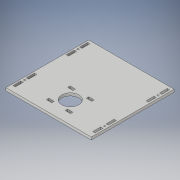
# Autodesk Inventor part: top
Saved by Autodesk Inventor 2018 (Build 220112000, 112)
## iProperties
Created: 2018-04-09
Part Number: top
Material: Generic
Document SubType Name: Modeling
Designer: guita
Density: 1 g/cm^3
Appearance: Default
Author: guita
Autodesk Inventor part; units mm, degrees
ref_plane "YZ Plane" through (0, 0, 0) normal (1, 0, 0) x (0, 1, 0)
ref_plane "XZ Plane" through (0, 0, 0) normal (0, 1, 0) x (-1, 0, 0)
ref_plane "XY Plane" through (0, 0, 0) normal (0, 0, 1) x (1, 0, 0)
sketch "Sketch1" plane through (0, 0, 0) normal (0, 1, 0) x (-1, 0, 0)
  line L0 (0, 0) -> (203.2, 0)
  line L1 (203.2, 0) -> (203.2, -196.85)
  line L2 (203.2, -196.85) -> (0, -196.85)
  line L3 (0, -196.85) -> (0, 0)
  line L4 (0, -196.85) -> (0, -190.5)
  line L5 (3.9624, -190.5) -> (9.525, -190.5)
  line L6 (9.525, -190.5) -> (9.525, -171.45)
  line L7 (9.525, -171.45) -> (3.9624, -171.45)
  circle A0 centre (6.35, -165.1) radius 1.9812
  line L8 (3.9624, -158.75) -> (9.525, -158.75)
  line L9 (9.525, -158.75) -> (9.525, -139.7)
  line L10 (9.525, -139.7) -> (3.9624, -139.7)
  line L11 (3.9624, -12.7) -> (9.525, -12.7)
  line L12 (9.525, -12.7) -> (9.525, -31.75)
  line L13 (9.525, -31.75) -> (3.9624, -31.75)
  circle A1 centre (6.35, -38.1) radius 1.9812
  line L14 (3.9624, -44.45) -> (9.525, -44.45)
  line L15 (9.525, -44.45) -> (9.525, -63.5)
  line L16 (9.525, -63.5) -> (3.9624, -63.5)
  line L17 (199.2376, -190.5) -> (193.675, -190.5)
  line L18 (193.675, -190.5) -> (193.675, -171.45)
  line L19 (193.675, -171.45) -> (199.2376, -171.45)
  circle A2 centre (196.85, -165.1) radius 1.9812
  line L20 (199.2376, -158.75) -> (193.675, -158.75)
  line L21 (193.675, -158.75) -> (193.675, -139.7)
  line L22 (193.675, -139.7) -> (199.2376, -139.7)
  line L23 (193.675, -63.5) -> (199.2376, -63.5)
  line L24 (193.675, -44.45) -> (193.675, -63.5)
  line L25 (199.2376, -44.45) -> (193.675, -44.45)
  circle A3 centre (196.85, -38.1) radius 1.9812
  line L26 (193.675, -12.7) -> (193.675, -31.75)
  line L27 (199.2376, -12.7) -> (193.675, -12.7)
  line L28 (193.675, -31.75) -> (199.2376, -31.75)
  line L29 (193.675, -63.5) -> (199.2376, -63.5)
  line L30 (199.2376, -63.5) -> (199.2376, -44.45)
  line L31 (199.2376, -44.45) -> (193.675, -44.45)
  line L32 (193.675, -44.45) -> (193.675, -63.5)
  line L33 (193.675, -31.75) -> (199.2376, -31.75)
  line L34 (199.2376, -31.75) -> (199.2376, -12.7)
  line L35 (199.2376, -12.7) -> (193.675, -12.7)
  line L36 (193.675, -12.7) -> (193.675, -31.75)
  line L37 (193.675, -139.7) -> (199.2376, -139.7)
  line L38 (199.2376, -139.7) -> (199.2376, -158.75)
  line L39 (199.2376, -158.75) -> (193.675, -158.75)
  line L40 (193.675, -158.75) -> (193.675, -139.7)
  line L41 (193.675, -171.45) -> (199.2376, -171.45)
  line L42 (199.2376, -171.45) -> (199.2376, -190.5)
  line L43 (199.2376, -190.5) -> (193.675, -190.5)
  line L44 (193.675, -190.5) -> (193.675, -171.45)
  line L45 (9.525, -12.7) -> (3.9624, -12.7)
  line L46 (3.9624, -12.7) -> (3.9624, -31.75)
  line L47 (3.9624, -31.75) -> (9.525, -31.75)
  line L48 (9.525, -31.75) -> (9.525, -12.7)
  line L49 (9.525, -44.45) -> (3.9624, -44.45)
  line L50 (3.9624, -44.45) -> (3.9624, -63.5)
  line L51 (3.9624, -63.5) -> (9.525, -63.5)
  line L52 (9.525, -63.5) -> (9.525, -44.45)
  line L53 (9.525, -139.7) -> (3.9624, -139.7)
  line L54 (3.9624, -139.7) -> (3.9624, -158.75)
  line L55 (3.9624, -158.75) -> (9.525, -158.75)
  line L56 (9.525, -158.75) -> (9.525, -139.7)
  line L57 (9.525, -171.45) -> (3.9624, -171.45)
  line L58 (3.9624, -171.45) -> (3.9624, -190.5)
  line L59 (3.9624, -190.5) -> (9.525, -190.5)
  line L60 (9.525, -190.5) -> (9.525, -171.45)
  point P0 (203.2, -190.5)
  dimension "d0" = 203.2
  dimension "d1" = 196.85
  dimension "d7" = 3.9624
  dimension "d9" = 19.05
  dimension "d34" = 5.5626
  dimension "d35" = 5.5626
  constraints: 122 end point, 16 parallel, 9 horizontal, 8 perpendicular, 7 point on line, 4 centre point
  measures "d0" distance of L1.end L2.end
  measures "d1" distance of L0.end L1.end
  measures "d7" diameter of A0
  measures "d9" distance of L9.end L8.end
  measures "d34" distance of L25.start L31.end
  measures "d35" distance of L13.end L47.end
extrude "Extrusion1" add sketch "Sketch1" along normal blind 6.35
sketch "Sketch2" plane through (0, 6.35, 0) normal (0, 1, 0) x (1, 0, 0)
  line L0 (-203.2, 196.85) -> (-203.2, 0) projected
  line L1 (-203.2, 0) -> (0, 0)
  line L2 (-203.2, 0) -> (0, 0) projected
  line L3 (-101.6, 0) -> (-101.6, 196.85)
  line L4 (0, 196.85) -> (-203.2, 196.85) projected
  line L5 (-101.6, 0) -> (-101.6, 29)
  line L6 (-101.6, 0) -> (-101.6, 103)
  line L7 (-101.6, 103) -> (-101.6, 74)
  line L8 (-101.6, 29) -> (-117.5512, 29)
  line L9 (-117.5512, 29) -> (-130.2512, 29)
  line L10 (-130.2512, 29) -> (-130.2512, 23.4374)
  line L11 (-117.5512, 23.4374) -> (-117.5512, 29)
  line L12 (-101.6, 74) -> (-117.5512, 74)
  line L13 (-117.5512, 74) -> (-130.2512, 74)
  line L14 (-130.2512, 74) -> (-130.2512, 79.5626)
  line L15 (-117.5512, 79.5626) -> (-117.5512, 74)
  line L16 (-101.6, 29) -> (-85.6488, 29)
  line L17 (-101.6, 74) -> (-85.6488, 74)
  line L18 (-85.6488, 29) -> (-72.9488, 29)
  line L19 (-72.9488, 29) -> (-72.9488, 23.4374)
  line L20 (-85.6488, 23.4374) -> (-85.6488, 29)
  line L21 (-85.6488, 74) -> (-72.9488, 74)
  line L22 (-72.9488, 74) -> (-72.9488, 79.5626)
  line L23 (-85.6488, 79.5626) -> (-85.6488, 74)
  line L24 (-101.6, 103) -> (-101.6, 72)
  line L25 (-101.6, 72) -> (-101.6, 51.5)
  circle A0 centre (-101.6, 51.5) radius 20.5
  line L26 (-130.2512, 29) -> (-117.5512, 29)
  line L27 (-117.5512, 29) -> (-117.5512, 23.4374)
  line L28 (-117.5512, 23.4374) -> (-130.2512, 23.4374)
  line L29 (-130.2512, 23.4374) -> (-130.2512, 29)
  line L30 (-85.6488, 29) -> (-72.9488, 29)
  line L31 (-72.9488, 29) -> (-72.9488, 23.4374)
  line L32 (-72.9488, 23.4374) -> (-85.6488, 23.4374)
  line L33 (-85.6488, 23.4374) -> (-85.6488, 29)
  line L34 (-130.2512, 74) -> (-117.5512, 74)
  line L35 (-117.5512, 74) -> (-117.5512, 79.5626)
  line L36 (-117.5512, 79.5626) -> (-130.2512, 79.5626)
  line L37 (-130.2512, 79.5626) -> (-130.2512, 74)
  line L38 (-85.6488, 74) -> (-72.9488, 74)
  line L39 (-72.9488, 74) -> (-72.9488, 79.5626)
  line L40 (-72.9488, 79.5626) -> (-85.6488, 79.5626)
  line L41 (-85.6488, 79.5626) -> (-85.6488, 74)
  dimension "d13" = 29
  dimension "d15" = 103
  dimension "d16" = 29
  dimension "d17" = 15.9512
  dimension "d20" = 15.9512
  dimension "d23" = 15.9512
  dimension "d29" = 31
  dimension "d30" = 20.5
  dimension "d31" = 41
  dimension "d37" = 5.5626
  constraints: 78 end point, 12 parallel, 11 perpendicular, 10 horizontal, 6 point on line, 3 midpoint, 1 centre point, 1 coincident
  measures "d13" distance of L3.start L5.end
  measures "d15" distance of L3.start L6.end
  measures "d16" distance of L6.end L7.end
  measures "d17" distance of L5.end L8.end
  measures "d20" distance of L7.end L12.end
  measures "d23" distance of L5.end L16.end
  measures "d29" distance of L6.end L24.end
  measures "d30" distance of L24.end L25.end
  measures "d31" diameter of A0
  measures "d37" distance of L15.start L34.end
extrude "Extrusion2" cut sketch "Sketch2" against normal blind 6.35 contours A0 L3 | L3 A0 | L11 L28 L10 L9 | L13 L14 L36 L15 | L18 L19 L32 L20 | L23 L40 L22 L21
body "Solid1"
